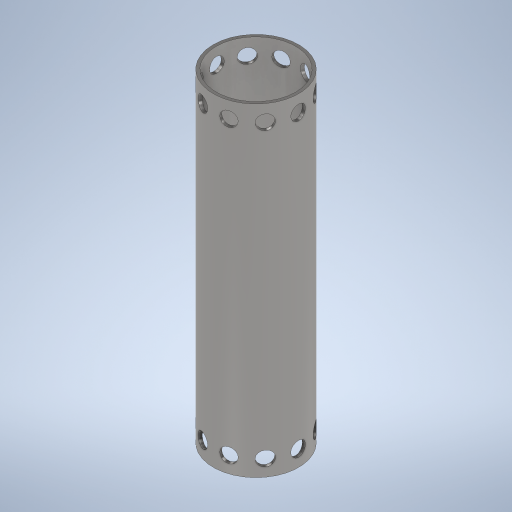
# Autodesk Inventor part: Metal_insert
Saved by Autodesk Inventor 2023 (Build 270158000, 158)
## iProperties
Created: 2022-09-20
Part Number: Metal_insert
Material: Сталь нержавеющая AISI 405
Document SubType Name: Modeling
Designer: Makar
Density: 8 g/cm^3
Appearance: С умеренной полировкой
Author: Makar
Autodesk Inventor part; units mm, degrees
ref_plane "YZ Plane" through (0, 0, 0) normal (1, 0, 0) x (0, 1, 0)
ref_plane "XZ Plane" through (0, 0, 0) normal (0, 1, 0) x (-1, 0, 0)
ref_plane "XY Plane" through (0, 0, 0) normal (0, 0, 1) x (1, 0, 0)
sketch "Эскиз1" plane through (0, 0, 0) normal (0, 1, 0) x (-1, 0, 0)
  circle A0 centre (0, 0) radius 13.5
  circle A1 centre (0, 0) radius 14.5
  dimension "d0" = 27
  dimension "d1" = 29
  constraints: 2 centre point, 2 coincident
  measures "d0" diameter of A0
  measures "d1" diameter of A1
extrude "Выдавливание1" add sketch "Эскиз1" along normal blind 110
sketch "Эскиз2" plane through (0, 0, 0) normal (1, 0, 0) x (0, 1, 0)
  line L0 (110, -14.5) -> (110, 14.5) projected
  line L1 (0, -14.5) -> (0, 14.5) projected
  line L2 (0, 14.5) -> (110, 14.5)
  line L3 (110, -14.5) -> (0, -14.5)
  circle A0 centre (5.5, 0) radius 2.5
  line L4 (55, 14.5) -> (55, -14.5)
  circle A1 centre (104.5, 0) radius 2.5
  point P0 (0, 0)
  dimension "d4" = 5
  dimension "d5" = 5.5
  constraints: 6 end point, 2 centre point, 2 midpoint, 1 horizontal, 1 parallel, 1 symmetric about line, 1 other
  measures "d4" diameter of A0
  measures "d5" distance from line of L1 A0.centre
extrude "Выдавливание2" cut sketch "Эскиз2" along normal mid plane 110 contours A0 | A1
pattern_circular "Круговой массив1" count 10 over 360 about axis through (0, 0, 0) along (0, 1, 0) of "Выдавливание2"
